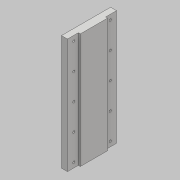
# Autodesk Inventor part: exercise3-14ipt
Saved by Autodesk Inventor 2018 (Build 220112000, 112)
## iProperties
Created: 2020-09-23
Part Number: exercise3-14ipt
Material: 一般
Document SubType Name: Modeling
Designer: 王鼎鈞
Density: 1 g/cm^3
Appearance: 預設
Author: 王鼎鈞
Autodesk Inventor part; units mm, degrees
ref_plane "YZ Plane" through (0, 0, 0) normal (1, 0, 0) x (0, 1, 0)
ref_plane "XZ Plane" through (0, 0, 0) normal (0, 1, 0) x (-1, 0, 0)
sketch "草圖1" plane through (0, 0, 0) normal (1, 0, 0) x (0, 1, 0)
  line L0 (-173.6, 0) -> (173.6, 0) projected
  line L1 (0, -406) -> (0, 406) projected
  line L2 (-124, 290) -> (124, 290)
  line L3 (124, 290) -> (124, -290)
  line L4 (124, -290) -> (-124, -290)
  line L5 (-124, -290) -> (-124, 290)
  line L6 (-124, 290) -> (124, -290) construction
  line L7 (124, 290) -> (-124, -290) construction
  point P0 (0, 0)
  dimension "d0" = 248
  dimension "d1" = 580
  constraints: 12 end point, 2 midpoint, 2 parallel, 1 horizontal, 1 perpendicular
  measures "d0" distance of L3.end L4.end
  measures "d1" distance of L2.end L3.end
extrude "擠出1" add sketch "草圖1" along normal blind 30
sketch "草圖2" plane through (30, 0, 0) normal (1, 0, 0) x (0, 0, -1)
  line L0 (-290, -69) -> (290, -69)
  line L1 (290, -69) -> (290, 69)
  line L2 (290, 69) -> (-290, 69)
  line L3 (-290, 69) -> (-290, -69)
  line L4 (-290, -69) -> (290, 69) construction
  line L5 (290, -69) -> (-290, 69) construction
  point P0 (0, 0)
  dimension "d4" = 580
  dimension "d5" = 138
  constraints: 12 end point, 2 midpoint, 2 parallel, 1 horizontal, 1 perpendicular
  measures "d4" distance of L2.end L1.end
  measures "d5" distance of L1.end L0.end
extrude "擠出2" add sketch "草圖2" along normal blind 10
sketch "草圖3" plane through (0, 0, 0) normal (-1, 0, 0) x (0, 0, 1)
  line L0 (0, -173.6) -> (0, 173.6) projected
  line L1 (-406, 0) -> (406, 0) projected
  line L2 (-290, 124) -> (-290, -124) projected
  point P0 (0, 0)
  point P1 (-265, 92)
  dimension "d8" = 92
  dimension "d9" = 25
  measures "d8" distance from line of L1 point (-265, 92)
  measures "d9" distance from line of L2 point (-265, 92)
hole "孔1" at (0, 92, -265) direction (1, 0, 0) diameter 11 end through all countersink diameter 12 countersink angle 90
delete faces "刪除面1" heal yes whole lump no faces at (0.1667, 86.1714, -265.2349)
chamfer "倒角1" distance 6 angle 45 1 edges at (0, 92, -270.5)
pattern_linear "矩形陣列1" count 5 spacing 132.5 along (0, 0, 1) of "孔1", "刪除面1", "倒角1"
ref_plane "工作平面1" through (30, 0, -290) normal (0, -1, 0) x (1, 0, 0)
mirror "鏡射1" about plane through (30, 0, -290) normal (0, -1, 0) of "孔1", "刪除面1", "倒角1", "矩形陣列1"
